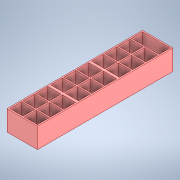
# Autodesk Inventor part: Contenedor2
Saved by Autodesk Inventor 2020.3 (Build 243373000, 373)
## iProperties
Created: 2020-08-31
Part Number: Contenedor2
Material: ABS Plastic
Document SubType Name: Modeling
Designer: juanp
Density: 1.06 g/cm^3
Appearance: Smooth - White
Author: juanp
Autodesk Inventor part; units mm, degrees
ref_plane "YZ Plane" through (0, 0, 0) normal (1, 0, 0) x (0, 1, 0)
ref_plane "XZ Plane" through (0, 0, 0) normal (0, 1, 0) x (-1, 0, 0)
ref_plane "XY Plane" through (0, 0, 0) normal (0, 0, 1) x (1, 0, 0)
sketch "Sketch1" plane through (0, 0, 0) normal (0, 0, 1) x (1, 0, 0)
  line L0 (-45, -30) -> (45, -30)
  line L1 (45, -30) -> (45, 30)
  line L2 (45, 30) -> (-45, 30)
  line L3 (-45, 30) -> (-45, -30)
  line L4 (-45, -30) -> (45, 30) construction
  line L5 (45, -30) -> (-45, 30) construction
  point P0 (0, 0)
  dimension "d0" = 90
  dimension "d1" = 60
  constraints: 12 end point, 2 midpoint, 2 parallel, 1 horizontal, 1 perpendicular
  measures "d0" distance of L2.end L1.end
  measures "d1" distance of L1.end L0.end
extrude "Extrusion1" add sketch "Sketch1" along normal blind 400
sketch "Sketch3" plane through (-45, 30, 0) normal (0, 1, 0) x (1, 0, 0)
  line L0 (4, -396) -> (43, -396)
  line L1 (43, -396) -> (43, -361)
  line L2 (43, -361) -> (4, -361)
  line L3 (4, -361) -> (4, -396)
  line L4 (90, -400) -> (0, -400) projected
  line L5 (0, 0) -> (0, -400) projected
  line L6 (47, -396) -> (86, -396)
  line L7 (86, -396) -> (86, -361)
  line L8 (86, -361) -> (47, -361)
  line L9 (47, -361) -> (47, -396)
  line L10 (90, 0) -> (90, -400) projected
  line L11 (4, -37) -> (86, -37)
  line L12 (86, -37) -> (86, -4)
  line L13 (86, -4) -> (4, -4)
  line L14 (4, -4) -> (4, -37)
  line L15 (90, 0) -> (0, 0) projected
  line L16 (43, -322) -> (4, -322)
  line L17 (4, -322) -> (4, -357)
  line L18 (4, -357) -> (43, -357)
  line L19 (43, -357) -> (43, -322)
  line L20 (47, -322) -> (47, -357)
  line L21 (86, -322) -> (47, -322)
  line L22 (47, -357) -> (86, -357)
  line L23 (86, -357) -> (86, -322)
  line L24 (43, -283) -> (4, -283)
  line L25 (4, -283) -> (4, -318)
  line L26 (4, -318) -> (43, -318)
  line L27 (43, -318) -> (43, -283)
  line L28 (47, -283) -> (47, -318)
  line L29 (86, -283) -> (47, -283)
  line L30 (47, -318) -> (86, -318)
  line L31 (86, -318) -> (86, -283)
  line L32 (43, -162) -> (4, -162)
  line L33 (4, -162) -> (4, -197)
  line L34 (4, -197) -> (43, -197)
  line L35 (47, -162) -> (47, -197)
  line L36 (43, -201) -> (4, -201)
  line L37 (4, -201) -> (4, -236)
  line L38 (4, -236) -> (43, -236)
  line L39 (86, -240) -> (47, -240)
  line L40 (43, -275) -> (43, -240)
  line L41 (4, -275) -> (43, -275)
  line L42 (43, -197) -> (43, -162)
  line L43 (86, -275) -> (86, -240)
  line L44 (4, -240) -> (4, -275)
  line L45 (43, -240) -> (4, -240)
  line L46 (47, -240) -> (47, -275)
  line L47 (47, -275) -> (86, -275)
  line L48 (86, -162) -> (47, -162)
  line L49 (86, -197) -> (86, -162)
  line L50 (43, -236) -> (43, -201)
  line L51 (47, -201) -> (47, -236)
  line L52 (47, -197) -> (86, -197)
  line L53 (86, -201) -> (47, -201)
  line L54 (86, -236) -> (86, -201)
  line L55 (47, -236) -> (86, -236)
  line L56 (43, -41) -> (4, -41)
  line L57 (4, -41) -> (4, -76)
  line L58 (4, -76) -> (43, -76)
  line L59 (47, -41) -> (47, -76)
  line L60 (43, -80) -> (4, -80)
  line L61 (4, -80) -> (4, -115)
  line L62 (4, -115) -> (43, -115)
  line L63 (86, -119) -> (47, -119)
  line L64 (43, -154) -> (43, -119)
  line L65 (4, -154) -> (43, -154)
  line L66 (43, -76) -> (43, -41)
  line L67 (86, -154) -> (86, -119)
  line L68 (4, -119) -> (4, -154)
  line L69 (43, -119) -> (4, -119)
  line L70 (47, -119) -> (47, -154)
  line L71 (47, -154) -> (86, -154)
  line L72 (86, -41) -> (47, -41)
  line L73 (86, -76) -> (86, -41)
  line L74 (43, -115) -> (43, -80)
  line L75 (47, -80) -> (47, -115)
  line L76 (47, -76) -> (86, -76)
  line L77 (86, -80) -> (47, -80)
  line L78 (86, -115) -> (86, -80)
  line L79 (47, -115) -> (86, -115)
  point P0 (45, 0)
  point P1 (0, -361)
  point P2 (90, -361)
  point P3 (0, -322)
  point P4 (90, -322)
  point P5 (0, -201)
  point P6 (0, -240)
  point P7 (0, -279)
  point P8 (90, -279)
  point P9 (90, -201)
  point P10 (90, -240)
  point P11 (0, -80)
  point P12 (0, -119)
  point P13 (0, -158)
  point P14 (90, -158)
  point P15 (90, -80)
  point P16 (90, -119)
  dimension "d4" = 4
  dimension "d7" = 4
  dimension "d9" = 35
  dimension "d19" = 4
  dimension "d20" = 4
  dimension "d21" = 4
  dimension "d38" = 4
  dimension "d39" = 4
  dimension "d41" = 4
  dimension "d44" = 39
  dimension "d51" = 121
  dimension "d56" = 4
  constraints: 152 end point, 6 parallel, 3 horizontal, 3 perpendicular, 2 equal length, 2 vertical, 144 other
  measures "d4" distance between parallel lines of L0 L4
  measures "d7" distance between parallel lines of L4 L6
  measures "d9" distance of L2.end L0.start
  measures "d19" distance between parallel lines of L5 L3
  measures "d20" distance between parallel lines of L10 L7
  measures "d21" distance between parallel lines of L9 L1
  measures "d38" distance between parallel lines of L12 L10
  measures "d39" distance between parallel lines of L5 L14
  measures "d41" distance between parallel lines of L15 L13
  measures "d44" distance of L2.end L16.end
  measures "d51" distance of L24.end L32.end
  measures "d56" distance between parallel lines of L11 L56
extrude "Extrusion2" cut sketch "Sketch3" against normal blind 56 contours L3 L2 L1 L0 | L9 L8 L7 L6 | L14 L13 L12 L11 | L19 L18 L17 L16 | L21 L23 L22 L20 | L27 L26 L25 L24 | L29 L31 L30 L28 | L42 L34 L33 L32 | L48 L49 L52 L35 | L50 L38 L37 L36 | L43 L47 L46 L39 | L41 L44 L45 L40 | L53 L54 L55 L51 | L66 L58 L57 L56 | L72 L73 L76 L59 | L74 L62 L61 L60 | L67 L71 L70 L63 | L65 L68 L69 L64 | L77 L78 L79 L75
ref_plane "Work Plane1" through (0, 0, 200) normal (0, 0, 1) x (1, 0, 0)
ref_plane "Work Plane2" through (0, -30, 0) normal (1, 0, 0) x (0, 0, -1)
body "Solid1"
